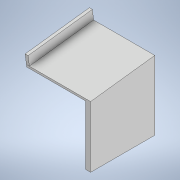
# Autodesk Inventor part: 斜面1
Saved by Autodesk Inventor 2020 (Build 240168000, 168)
## iProperties
Created: 2020-12-07
Part Number: 斜面1
Material: 常规
Document SubType Name: Sheet Metal
Designer: huang
Density: 1 g/cm^3
Sheet Metal Rule: 默认_mm
Appearance: 默认
Author: huang
Autodesk Inventor part; units mm, degrees
ref_plane "YZ Plane" through (0, 0, 0) normal (1, 0, 0) x (0, 1, 0)
ref_plane "XZ Plane" through (0, 0, 0) normal (0, 1, 0) x (-1, 0, 0)
ref_plane "XY Plane" through (0, 0, 0) normal (0, 0, 1) x (1, 0, 0)
sketch "草图1" plane through (0, 0, 0) normal (0, 1, 0) x (-1, 0, 0)
  line L0 (0, 0) -> (65, 0)
  line L1 (65, 0) -> (65, -65)
  line L2 (65, -65) -> (0, -65)
  line L3 (0, -65) -> (0, 0)
  dimension "d0" = 65
  dimension "d1" = 65
  constraints: 8 end point, 2 parallel, 1 horizontal, 1 perpendicular
  measures "d0" distance of L0.end L1.end
  measures "d1" distance of L1.end L2.end
extrude "拉伸1" add sketch "草图1" along normal blind 10
chamfer "倒角1" distance 65 angle 7 1 edges at (-32.5, 10, 0) measured on face at (-32.5, 10, -0.5)
sketch "草图2" plane through (0, 0, 0) normal (0, -1, 0) x (1, 0, 0)
  line L0 (-65, 0) -> (0, 0) projected
  line L1 (-32.5, 0) -> (-32.5, -65)
  line L2 (0, -65) -> (-65, -65) projected
  circle A0 centre (-32.5, -32.5) radius 1.95
  dimension "d7" = 3.9
  constraints: 3 midpoint, 2 end point, 1 centre point
  measures "d7" diameter of A0
extrude "拉伸2" cut sketch "草图2" against normal blind 4
sketch "草图4" plane through (0, 0, 0) normal (0, -1, 0) x (1, 0, 0)
  line L0 (0, 0) -> (0, -65) projected
  line L1 (0, -65) -> (-65, -65) projected
  line L2 (0, 0) -> (-5, 0)
  line L3 (-5, 0) -> (-5, -65)
  line L4 (-5, -65) -> (0, -65)
  line L5 (0, -65) -> (0, 0)
  dimension "d13" = 5
  constraints: 8 end point, 2 parallel, 1 horizontal, 1 perpendicular, 1 point on line
  measures "d13" distance between parallel lines of L3 L0
extrude "拉伸4" add sketch "草图4" along normal blind 60
sketch "草图5" plane through (-65, 10, -65) normal (0, 0.9925462, 0.1218693) x (1, 0, 0)
  line L0 (0, 0) -> (3, 0)
  line L1 (3, 0) -> (3, -35.2725)
  line L2 (3, -35.2725) -> (0, -35.2725)
  line L3 (0, -35.2725) -> (0, 0)
  line L4 (0, -65.4881) -> (65, -65.4881) projected
  line L5 (0, 0) -> (3, 0)
  line L6 (3, 0) -> (3, -65.4881)
  line L7 (3, -65.4881) -> (0, -65.4881)
  line L8 (0, -65.4881) -> (0, 0)
  point P0 (65, -65.7342)
  point P1 (0, -35.2725)
  point P2 (0, -65.4881)
  point P3 (3, -35.2725)
  dimension "d17" = 3
  constraints: 16 end point, 4 parallel, 2 horizontal, 2 perpendicular, 1 point on line
  measures "d17" distance between parallel lines of L1 L3
extrude "拉伸5" add sketch "草图5" along normal blind 10
equation "\"折弯半径\" = 厚度"
equation "\"折弯释压宽度\" = 厚度"
equation "\"折弯释压深度\" = 0.5 * 厚度"
equation "\"拐角释压尺寸\" = 4 * 厚度"
equation "\"最小余量\" = 2 * 厚度"
equation "\"过渡半径\" = 折弯半径"
equation "\"Jacobi半径尺寸\" = 折弯半径"
equation "\"间隙大小\" = 厚度"
equation "\"厚度\" = 0.5"
